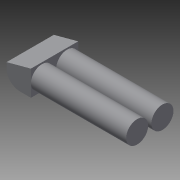
# Autodesk Inventor part: DMJ_Legs
Saved by Autodesk Inventor 2015 SP1 (Build 190203100, 203)
## iProperties
Created: 2016-02-03
Part Number: DMJ_Legs
Material: Generic
Document SubType Name: Modeling
Designer: guillemd
Density: 0.665801 g/cm^3
Appearance: Default
Mass: 31751.5 g
Surface Area: 11536.8 cm^2
Volume: 47689.2 cm^3
Author: guillemd
Autodesk Inventor part; units mm, degrees
ref_plane "YZ Plane" through (0, 0, 0) normal (1, 0, 0) x (0, 1, 0)
ref_plane "XZ Plane" through (0, 0, 0) normal (0, 1, 0) x (-1, 0, 0)
ref_plane "XY Plane" through (0, 0, 0) normal (0, 0, 1) x (1, 0, 0)
sketch "Sketch1" plane through (0, 0, 0) normal (0, 0, 1) x (1, 0, 0)
  line L0 (0, 203.2) -> (0, 0)
  line L1 (0, 0) -> (-88.9, 0)
  line L2 (-196.2761, 150.608) -> (-196.2761, 107.3761)
  arc A0 (-196.2761, 107.3761) -> (-88.9, 0) centre (-88.9, 107.3761) ccw
  line L3 (-196.2761, 150.608) -> (0, 203.2)
  line L4 (0, -67.326) -> (0, 248.2877) projected
  dimension "d1" = 203.2
  dimension "d2" = 75
  dimension "d3" = 203.2
  dimension "d4" = 88.9
  constraints: 8 end point, 2 perpendicular, 2 point on circle, 2 tangent, 1 centre point, 1 coincident, 1 horizontal, 1 point on line
  measures "d1" distance of L0.start L2.start
  measures "d2" angle of L0 L3
  measures "d3" distance of L0.start L0.end
  measures "d4" horizontal distance of point (0, 0) A0.centre
extrude "Extrusion1" add sketch "Sketch1" along normal mid plane 381
sketch "Sketch2" plane through (0, 0, 190.5) normal (1, 0, 0) x (0, 0, -1)
  circle A0 centre (88.9, 101.6) radius 88.9
  circle A1 centre (292.2878, 101.6) radius 88.9
  line L0 (381, 203.2) -> (0, 203.2) projected
  line L1 (0, 0) -> (0, 203.2)
  line L2 (381, 203.2) -> (381, 0)
  point P0 (190.5, 0)
  point P1 (0, 150.608)
  point P2 (366.6135, 150.374)
  point P3 (381, 0)
  point P4 (381, 107.3761)
  point P5 (0, 101.6)
  dimension "d7" = 177.8
  dimension "d8" = 177.8
  dimension "d16" = 101.6
  dimension "d17" = 101.6
  constraints: 2 end point, 2 point on circle, 1 centre point, 1 coincident, 1 horizontal alignment, 1 midpoint, 5 other
  measures "d8" diameter of A1
  measures "d16" distance from line of L0 point (88.9, 101.6)
  measures "d17" distance from line of A1.centre L0
extrude "Extrusion2" add sketch "Sketch2" along normal blind 767.08
body "Solid1"
